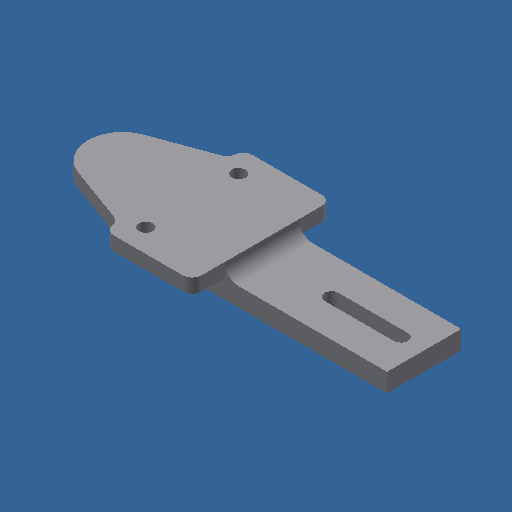
# Autodesk Inventor part: Acople_sensor_hall
Saved by Autodesk Inventor 2025 (Build 290162000, 162)
## iProperties
Created: 2025-09-16
Part Number: Acople_sensor_hall
Material: Generic
Document SubType Name: Modeling
Designer: HP
Density: 1 g/cm^3
Appearance: Default
Author: HP
Autodesk Inventor part; units mm, degrees
ref_plane "Plano de trabajo1" through (10, 0, 0) normal (1, 0, 0) x (0, 1, 0)
ref_plane "XZ Plane" through (0, 0, 0) normal (0, 1, 0) x (-1, 0, 0)
ref_plane "XY Plane" through (0, 0, 0) normal (0, 0, 1) x (1, 0, 0)
sketch "Boceto6" plane through (0, 0, 0) normal (0, 1, 0) x (-1, 0, 0)
  circle A0 centre (0, 0) radius 7.5
  dimension "d24" = 15
  constraints: 1 centre point, 1 coincident
  measures "d24" diameter of A0
extrude "Extrusión6" add sketch "Boceto6" along normal blind 3
sketch "Boceto7" plane through (0, 0, 0) normal (0, 1, 0) x (-1, 0, 0)
  circle A0 centre (0, 0) radius 7.5 projected
  line L0 (2.5652, 7.0477) -> (-11.0412, 12)
  line L1 (-11.0412, 12) -> (-11.0412, 15)
  line L2 (-11.0412, 15) -> (-17.2417, 15)
  line L3 (-17.2417, 15) -> (-27.2111, 15)
  line L4 (-27.2111, 15) -> (-30, 15)
  line L5 (-30, 15) -> (-30, 0)
  line L6 (0, 0) -> (-21.4903, 0) construction
  line L7 (2.5652, -7.0477) -> (-11.0412, -12)
  line L8 (-11.0412, -12) -> (-11.0412, -15)
  line L9 (-11.0412, -15) -> (-17.2417, -15)
  line L10 (-17.2417, -15) -> (-27.2111, -15)
  line L11 (-27.2111, -15) -> (-30, -15)
  line L12 (-30, -15) -> (-30, 0)
  point P0 (2.5652, -7.0477)
  dimension "d28" = 110
  dimension "d29" = 3
  dimension "d30" = 30
  dimension "d31" = 15
  constraints: 26 end point, 6 symmetric about line, 4 point on line, 2 horizontal, 2 perpendicular, 3 other
  measures "d28" angle of L0 L1
  measures "d29" distance of L0.end L1.end
  measures "d30" distance from line of point (0, 0) L5
  measures "d31" distance between parallel lines of L3 L6
extrude "Extrusión7" add sketch "Boceto7" along normal blind 3 contours A0 L7 L8 L9 L10 L11 L12 L5 L4 L3 L2 L1 L0
sketch "Boceto8" plane through (0, 3, 0) normal (0, 1, 0) x (1, 0, 0)
  line L0 (11.0412, -15) -> (30, -15) projected
  line L1 (30, -15) -> (30, 15) projected
  line L2 (30, 15) -> (11.0412, 15) projected
  line L3 (13.522, 10) -> (35, 10) construction
  circle A0 centre (15, 10) radius 1.5
  line L4 (0, 0) -> (26.0332, 0) construction
  circle A1 centre (15, -10) radius 1.5
  dimension "d35" = 5
  dimension "d36" = 3
  dimension "d37" = 15
  constraints: 4 end point, 2 centre point, 1 horizontal, 1 point on line, 1 symmetric about line, 1 other
  measures "d35" distance between parallel lines of L3 L2
  measures "d36" diameter of A0
  measures "d37" horizontal distance of A0.centre L4.start
extrude "Extrusión8" cut sketch "Boceto8" against normal blind 3
fillet "Empalme1" radius 2 4 edges at (11.0412, 1.5, -12) (11.0412, 1.5, 12) (11.0412, 1.5, 15) (11.0412, 1.5, -15)
fillet "Empalme2" radius 2 2 edges at (30, 1.5, -15) (30, 1.5, 15)
sketch "Boceto9" plane through (0, 0, 0) normal (0, -1, 0) x (1, 0, 0)
  line L0 (25, -8) -> (65, -8)
  line L1 (65, -8) -> (65, 8)
  line L2 (65, 8) -> (25, 8)
  line L3 (25, 8) -> (25, -8)
  line L4 (0, 0) -> (25, 0) construction
  line L5 (45, 0) -> (60, 0)
  line L6 (45, -1.5) -> (60, -1.5)
  line L7 (60, 1.5) -> (45, 1.5)
  arc A0 (45, 1.5) -> (45, -1.5) centre (45, 0) ccw
  arc A1 (60, -1.5) -> (60, 1.5) centre (60, 0) ccw
  point P0 (52.5, 0)
  point P1 (25, 0)
  dimension "d42" = 40
  dimension "d43" = 16
  dimension "d44" = 25
  dimension "d45" = 8
  dimension "d46" = 3
  dimension "d47" = 15
  dimension "d48" = 20
  constraints: 18 end point, 4 point on circle, 4 tangent, 3 midpoint, 3 parallel, 2 centre point, 2 horizontal, 2 perpendicular, 1 horizontal alignment
  measures "d42" distance of L2.end L1.end
  measures "d43" distance of L1.end L0.end
  measures "d44" distance of L4.start L4.end
  measures "d45" distance between parallel lines of L4 L0
  measures "d46" diameter of A1
  measures "d47" distance of L7.start L7.end
  measures "d48" distance of point (25, 0) L5.start
extrude "Extrusión9" add sketch "Boceto9" along normal blind 4
fillet "Empalme3" radius 3 2 edges at (30, 0, 0) (25, 0, 0)
sketch "Boceto1" plane through (0, 0, 0) normal (0, 1, 0) x (-1, 0, 0)
  circle A0 centre (0, 0) radius 10
  circle A1 centre (0, 0) radius 7.5
  dimension "d0" = 20
  dimension "d1" = 15
  constraints: 2 centre point, 2 coincident
  measures "d0" diameter of A0
  measures "d1" diameter of A1
sketch "Boceto2" plane through (0, 0, 0) normal (0, -1, 0) x (1, 0, 0)
  circle A0 centre (0, 0) radius 10 projected
sketch "Boceto4" plane through (10, 0, 0) normal (1, 0, 0) x (0, 1, 0)
  line L0 (-4, -10) -> (5, -10) projected
  line L1 (-4, 10) -> (-4, -10) projected
  line L2 (-4, 10) -> (5, 10) projected
  line L3 (5, -10) -> (5, 10) projected
  line L4 (0, 7.5) -> (0, -7.5) projected
  line L5 (-1.1, -7.5) -> (-2.9, -7.5)
  line L6 (-2.9, -7.5) -> (-2.9, 7.5)
  line L7 (-2.9, 7.5) -> (-1.1, 7.5)
  line L8 (-1.1, 7.5) -> (-1.1, -7.5)
  point P0 (0, 0)
  point P1 (-2, -7.5)
  dimension "d7" = 1.8
  dimension "d8" = 15
  dimension "d9" = 2.5
  dimension "d10" = 1.1
  dimension "d13" = 2
  dimension "d16" = 4
  dimension "d17" = 1.5
  dimension "d19" = 2.5
  constraints: 3 centre point, 2 end point, 1 coincident, 1 midpoint, 1 symmetric about line, 2 other
